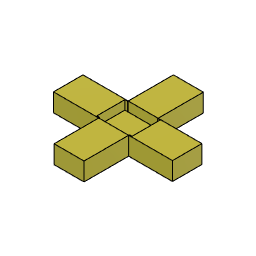
BMO_Joystick (Autodesk Fusion 360 design; units mm, degrees)
Autodesk Fusion 360 part; units mm, degrees
sketch "스케치1" plane through (0, 0, 0) normal (0, 1, 0) x (1, 0, 0)
  line L0 (5.2558, 0.4095) -> (68.4042, 0.4095)
  line L1 (73.4042, -4.5905) -> (73.4042, -43.5505)
  line L2 (0.2558, -43.5505) -> (0.2558, -4.5905)
  arc A0 (5.2558, 0.4095) -> (0.2558, -4.5905) centre (5.2558, -4.5905) ccw
  arc A1 (0.2558, -43.5505) -> (5.2558, -48.5505) centre (5.2558, -43.5505) ccw
  arc A2 (73.4042, -4.5905) -> (68.4042, 0.4095) centre (68.4042, -4.5905) ccw
  arc A3 (68.4259, -48.5505) -> (73.4042, -43.5505) centre (68.4042, -43.5505) ccw
  line L3 (8.0983, -61.4076) -> (32.8013, -61.4076)
  line L4 (32.8013, -61.4076) -> (32.8013, -65.2763)
  line L5 (32.8013, -65.2763) -> (8.0983, -65.2763)
  line L6 (8.0983, -65.2763) -> (8.0983, -61.4076)
  line L7 (33.6828, -66.6579) -> (7.2167, -66.6579)
  line L8 (6.7167, -66.1579) -> (6.7167, -60.526)
  line L9 (7.2167, -60.026) -> (33.6828, -60.026)
  line L10 (34.1828, -60.526) -> (34.1828, -66.1579)
  arc A4 (7.2167, -60.026) -> (6.7167, -60.526) centre (7.2167, -60.526) ccw
  arc A5 (6.7167, -66.1579) -> (7.2167, -66.6579) centre (7.2167, -66.1579) ccw
  arc A6 (34.1828, -60.526) -> (33.6828, -60.026) centre (33.6828, -60.526) ccw
  arc A7 (33.6828, -66.6579) -> (34.1828, -66.1579) centre (33.6828, -66.1579) ccw
  line L11 (19.1249, -96.9501) -> (32.2249, -96.9501)
  line L12 (32.2249, -96.9501) -> (32.2249, -102.6301)
  line L13 (32.2249, -102.6301) -> (19.1249, -102.6301)
  line L14 (19.1249, -102.6301) -> (19.1249, -96.9501)
  line L15 (3.6186, -96.8594) -> (16.7186, -96.8594)
  line L16 (16.7186, -96.8594) -> (16.7186, -102.5394)
  line L17 (16.7186, -102.5394) -> (3.6186, -102.5394)
  line L18 (3.6186, -102.5394) -> (3.6186, -96.8594)
  line L19 (-5.4373, 16.7169) -> (79.6514, 16.7169)
  line L20 (81.6514, 14.7169) -> (81.6514, -111.2831)
  line L21 (79.6514, -113.2831) -> (-5.4373, -113.2831)
  line L22 (-7.4373, -111.2831) -> (-7.4373, 14.7169)
  line L23 (12.7325, -76.8859) -> (16.6325, -76.8859)
  line L24 (16.6325, -76.8859) -> (16.6325, -79.9859)
  line L25 (16.6325, -79.9859) -> (12.7325, -79.9859)
  line L26 (12.7325, -79.9859) -> (12.7325, -76.8859)
  circle A8 centre (57.8034, -66.7955) radius 7
  circle A9 centre (56.6109, -95.955) radius 13.4
  circle A10 centre (56.6109, -95.955) radius 12
  line L27 (13.0415, -71.8299) -> (16.3471, -71.8299)
  line L28 (16.3471, -71.8299) -> (16.3471, -85.0178)
  line L29 (16.3471, -85.0178) -> (13.0415, -85.0178)
  line L30 (13.0415, -85.0178) -> (13.0415, -71.8299)
  line L31 (8.0415, -76.8299) -> (21.1916, -76.8299)
  line L32 (21.1916, -76.8299) -> (21.1916, -80.0863)
  line L33 (21.1916, -80.0863) -> (8.0415, -80.0863)
  line L34 (8.0415, -80.0863) -> (8.0415, -76.8299)
  line L35 (6.7208, -81.407) -> (6.7208, -75.5092)
  line L36 (6.7208, -75.5092) -> (22.5123, -75.5092)
  line L37 (22.5123, -75.5092) -> (22.5123, -81.407)
  line L38 (22.5123, -81.407) -> (6.7208, -81.407)
  line L39 (11.7155, -86.3438) -> (11.7155, -70.5039)
  line L40 (11.7155, -70.5039) -> (17.6731, -70.5039)
  line L41 (17.6731, -70.5039) -> (17.6731, -86.3438)
  line L42 (17.6731, -86.3438) -> (11.7155, -86.3438)
  arc A11 (-5.4373, 16.7169) -> (-7.4373, 14.7169) centre (-5.4373, 14.7169) ccw
  arc A12 (-3.4468, 14.3074) -> (-5.4468, 12.3074) centre (-3.4468, 12.3074) ccw
  arc A13 (81.6514, 14.7169) -> (79.6514, 16.7169) centre (79.6514, 14.7169) ccw
  arc A14 (79.6419, 12.3074) -> (77.6419, 14.3074) centre (77.6419, 12.3074) ccw
  arc A15 (-7.4373, -111.2831) -> (-5.4373, -113.2831) centre (-5.4373, -111.2831) ccw
  arc A16 (-5.4468, -102.8328) -> (-3.4468, -104.8328) centre (-3.4468, -102.8328) ccw
  arc A17 (77.6419, -104.8328) -> (79.6419, -102.8328) centre (77.6419, -102.8328) ccw
  arc A18 (79.6514, -113.2831) -> (81.6514, -111.2831) centre (79.6514, -111.2831) ccw
  line L43 (79.6514, 14.7169) -> (79.6514, -111.2831)
  line L44 (-5.4373, 14.7169) -> (79.6514, 14.7169)
  line L45 (-5.4373, -111.2831) -> (-5.4373, 14.7169)
  line L46 (79.6514, -111.2831) -> (-5.4373, -111.2831)
  line L47 (42.3168, -54.3547) -> (72.3168, -54.3547)
  line L48 (72.3168, -54.3547) -> (72.3168, -79.8547)
  line L49 (72.3168, -79.8547) -> (42.3168, -79.8547)
  line L50 (42.3168, -79.8547) -> (42.3168, -54.3547)
  arc A19 (-1.2442, -43.5505) -> (5.2558, -50.0505) centre (5.2558, -43.5505) ccw
  line L51 (-1.2442, -43.5505) -> (-1.2442, -4.5905)
  arc A20 (5.2558, 1.9095) -> (-1.2442, -4.5905) centre (5.2558, -4.5905) ccw
  line L52 (5.2558, 1.9095) -> (68.4042, 1.9095)
  arc A21 (74.9042, -4.5905) -> (68.4042, 1.9095) centre (68.4042, -4.5905) ccw
  line L53 (74.9042, -4.5905) -> (74.9042, -43.5505)
  arc A22 (68.4323, -50.0505) -> (74.9042, -43.5505) centre (68.4042, -43.5505) ccw
  line L54 (5.2558, -50.0505) -> (68.4323, -50.0505)
  line L55 (5.2558, -48.5505) -> (68.4259, -48.5505)
  line L56 (-3.5681, -64.3856) -> (30.2319, -64.3856)
  line L57 (30.2319, -64.3856) -> (30.2319, -91.3856)
  line L58 (30.2319, -91.3856) -> (-3.5681, -91.3856)
  line L59 (-3.5681, -91.3856) -> (-3.5681, -64.3856)
  line L60 (3.782, -65.3602) -> (24.782, -65.3602)
  line L61 (24.782, -65.3602) -> (24.782, -91.2602)
  line L62 (24.782, -91.2602) -> (3.782, -91.2602)
  line L63 (3.782, -91.2602) -> (3.782, -65.3602)
  point P0 (-7.4373, 16.7169)
  point P1 (81.6514, 16.7169)
  point P2 (81.6514, -113.2831)
  point P3 (-5.4468, 14.3074)
  point P4 (79.6419, 14.3074)
  point P5 (79.6419, -104.8328)
  dimension "d3" = 5
  dimension "d4" = 5
  dimension "d5" = 5
  dimension "d6" = 5
  dimension "d10" = 0.5
  dimension "d11" = 0.5
  dimension "d12" = 0.5
  dimension "d13" = 0.5
  dimension "d14" = 13.1
  dimension "d15" = 5.68
  dimension "d16" = 13.1
  dimension "d17" = 5.68
  dimension "d20" = 89.0887
  dimension "d21" = 130
  dimension "d22" = 85.0887
  dimension "d23" = 119.1403
  dimension "d24" = 26.4662
  dimension "d25" = 5.6319
  dimension "d26" = 24.703
  dimension "d27" = 3.8687
  dimension "d28" = 63.1484
  dimension "d29" = 38.96
  dimension "d32" = 3.9
  dimension "d33" = 3.1
  dimension "d34" = 14
  dimension "d35" = 26.8
  dimension "d36" = 24
  dimension "d37" = -1.3207
  dimension "d38" = -1.326
  dimension "d39" = 13.1501
  dimension "d40" = 15.7915
  dimension "d41" = 3.3056
  dimension "d42" = 15.8399
  dimension "d43" = 13.1879
  dimension "d44" = 3.2564
  dimension "d45" = 5.8978
  dimension "d46" = 2
  dimension "d47" = 2
  dimension "d48" = 2
  dimension "d49" = 2
  dimension "d50" = 2
  dimension "d51" = 2
  dimension "d52" = 2
  dimension "d53" = 2
  dimension "d54" = 14.8074
  dimension "d57" = 2
  dimension "d95" = 30
  dimension "d96" = 25.5
  dimension "d119" = 33.8
  dimension "d120" = 27
  dimension "d121" = 21
  dimension "d122" = 25.9
  constraint horizontal L0
  constraint vertical L1
  constraint vertical L2
  constraint tangent L2 A0
  constraint tangent L0 A0
  constraint tangent L2 A1
  constraint tangent L1 A2
  constraint tangent L0 A2
  constraint tangent L1 A3
  constraint horizontal L3
  constraint vertical L4
  constraint horizontal L5
  constraint vertical L6
  constraint parallel L5 L7
  constraint parallel L6 L8
  constraint parallel L3 L9
  constraint parallel L4 L10
  constraint tangent L8 A4
  constraint tangent L9 A4
  constraint tangent L8 A5
  constraint tangent L7 A5
  constraint tangent L9 A6
  constraint tangent L10 A6
  constraint tangent L10 A7
  constraint tangent L7 A7
  constraint horizontal L11
  constraint vertical L12
  constraint horizontal L13
  constraint vertical L14
  constraint horizontal L15
  constraint vertical L16
  constraint horizontal L17
  constraint vertical L18
  constraint horizontal L19
  constraint vertical L20
  constraint horizontal L21
  constraint vertical L22
  constraint horizontal L23
  constraint vertical L24
  constraint horizontal L25
  constraint vertical L26
  constraint concentric A9 A10
  constraint horizontal L27
  constraint vertical L28
  constraint horizontal L29
  constraint vertical L30
  constraint horizontal L31
  constraint vertical L32
  constraint horizontal L33
  constraint vertical L34
  constraint coincident P0 L22
  constraint coincident P0 L19
  constraint tangent L22 A11
  constraint tangent L19 A11
  constraint coincident P1 L19
  constraint coincident P1 L20
  constraint tangent L19 A13
  constraint tangent L20 A13
  constraint tangent L22 A15
  constraint tangent L21 A15
  constraint coincident P2 L20
  constraint coincident P2 L21
  constraint tangent L20 A18
  constraint tangent L21 A18
  constraint horizontal L47
  constraint vertical L48
  constraint horizontal L49
  constraint vertical L50
  constraint concentric A1 A19
  constraint parallel L2 L51
  constraint concentric A0 A20
  constraint parallel L0 L52
  constraint concentric A2 A21
  constraint parallel L1 L53
  constraint concentric A3 A22
  constraint tangent L52 A21
  constraint tangent A19 L51
  constraint tangent L53 A22
  constraint tangent A21 L53
  constraint tangent L51 A20
  constraint tangent A20 L52
  constraint horizontal L56
  constraint vertical L57
  constraint horizontal L58
  constraint vertical L59
  constraint horizontal L60
  constraint vertical L61
  constraint horizontal L62
  constraint vertical L63
  measures "d3" radius of A0
  measures "d4" radius of A1
  measures "d5" radius of A2
  measures "d6" radius of A3
  measures "d10" radius of A4
  measures "d11" radius of A5
  measures "d12" radius of A6
  measures "d13" radius of A7
  measures "d14" distance of L11.start L11.end
  measures "d15" distance of L11.start L13.end
  measures "d16" distance of L15.start L15.end
  measures "d17" distance of L15.start L17.end
  measures "d20" distance of P0 P1
  measures "d21" distance of P1 P2
  measures "d22" distance of P3 P4
  measures "d23" distance of P4 P5
  measures "d24" distance of L9.start L9.end
  measures "d25" distance of L10.start L10.end
  measures "d26" distance of L3.start L3.end
  measures "d27" distance of L3.end L4.end
  measures "d28" distance of A20.start L52.end
  measures "d29" distance of A21.start L53.end
  measures "d32" distance of L23.start L23.end
  measures "d33" distance of L23.start L25.end
  measures "d34" diameter of A8
  measures "d35" diameter of A9
  measures "d36" diameter of A10
  measures "d39" distance of L31.start L31.end
  measures "d40" distance of L35.end L36.end
  measures "d41" distance of L27.start L27.end
  measures "d42" distance of L39.start L39.end
  measures "d43" distance of L27.start L29.end
  measures "d44" distance of L31.start L33.end
  measures "d45" distance of L35.start L35.end
  measures "d46" radius of A11
  measures "d47" radius of A12
  measures "d48" radius of A13
  measures "d49" radius of A14
  measures "d50" radius of A15
  measures "d51" radius of A16
  measures "d52" radius of A17
  measures "d53" radius of A18
  measures "d54" distance of L19 L52
  measures "d95" distance of L48.end L49.end
  measures "d96" distance of L47.end L48.end
  measures "d119" distance of L56.start L56.end
  measures "d120" distance of L56.start L58.end
  measures "d121" distance of L60.start L60.end
  measures "d122" distance of L60.start L62.end
sketch "스케치2" plane through (286.6514, 0, 0) normal (1, 0, 0) x (0, 0, -1)
  line L0 (-111.2831, 0) -> (14.7169, 0)
  line L1 (14.7169, 0) -> (14.7169, 30)
  line L2 (14.7169, 30) -> (-111.2831, 30)
  line L3 (-111.2831, 30) -> (-111.2831, 0)
  line L4 (-87.1899, 4.8048) -> (5.0207, 5.1018) construction
  line L5 (5.0207, 5.1018) -> (4.9496, 27.1657) construction
  line L6 (4.9496, 27.1657) -> (-87.261, 26.8686) construction
  line L7 (-87.261, 26.8686) -> (-87.1899, 4.8048) construction
  circle A0 centre (-98, 14) radius 1
  circle A1 centre (-94.5923, 21.5266) radius 1
  circle A2 centre (-105.6179, 15.0752) radius 1
  circle A3 centre (-101.4738, 8.3604) radius 1
  circle A4 centre (-93.909, 8.4262) radius 1
  circle A5 centre (-91.1462, 14.9435) radius 1
  circle A6 centre (-101.408, 21) radius 1
  dimension "d74" = 25
  dimension "d84" = 2
  dimension "d85" = 2
  dimension "d87" = 2
  dimension "d88" = 2
  dimension "d89" = 2
  dimension "d90" = 2
  dimension "d91" = 2
  measures "d84" diameter of A0
  measures "d85" diameter of A1
  measures "d87" diameter of A2
  measures "d88" diameter of A3
  measures "d89" diameter of A4
  measures "d90" diameter of A5
  measures "d91" diameter of A6
sketch "스케치3" plane through (197.5627, 0, 0) normal (-1, 0, 0) x (0, 0, 1)
  line L0 (-14.7169, 0) -> (111.2831, 0)
  line L1 (111.2831, 0) -> (111.2831, 30)
  line L2 (111.2831, 30) -> (-14.7169, 30)
  line L3 (-14.7169, 30) -> (-14.7169, 0)
  line L4 (7.2946, 2.9984) -> (75.3904, 3.0024) construction
  line L5 (75.3904, 3.0024) -> (75.389, 27.1757) construction
  line L6 (75.389, 27.1757) -> (7.2931, 27.1717) construction
  line L7 (7.2931, 27.1717) -> (7.2946, 2.9984) construction
  dimension "d77" = 25
sketch "스케치4" plane through (0, 2, 0) normal (0, 1, 0) x (-1, 0, 0)
  arc A0 (-92.5627, 111.2831) -> (-94.5627, 113.2831) centre (-94.5627, 111.2831) ccw
  line L0 (-94.5627, 113.2831) -> (-179.6514, 113.2831)
  arc A1 (-179.6514, 113.2831) -> (-181.6514, 111.2831) centre (-179.6514, 111.2831) ccw
  line L1 (-181.6514, 111.2831) -> (-181.6514, -14.7169)
  arc A2 (-181.6514, -14.7169) -> (-179.6514, -16.7169) centre (-179.6514, -14.7169) ccw
  line L2 (-179.6514, -16.7169) -> (-94.5627, -16.7169)
  arc A3 (-94.5627, -16.7169) -> (-92.5627, -14.7169) centre (-94.5627, -14.7169) ccw
  line L3 (-92.5627, -14.7169) -> (-92.5627, 111.2831)
  line L4 (-104.1542, -7.6516) -> (-110, -7.6516)
  line L5 (-110, -7.6516) -> (-110, 25)
  line L6 (-110, 25) -> (-104.1542, 25)
  line L7 (-104.1542, 25) -> (-104.1542, -7.6516)
  line L8 (-126, -7.6516) -> (-126, 25)
  line L9 (-120.1542, 25) -> (-120.1542, -7.6516)
  line L10 (-126, 25) -> (-120.1542, 25)
  line L11 (-120.1542, -7.6516) -> (-126, -7.6516)
  line L12 (-141, -7.6516) -> (-141, 25)
  line L13 (-135.1542, 25) -> (-135.1542, -7.6516)
  line L14 (-141, 25) -> (-135.1542, 25)
  line L15 (-135.1542, -7.6516) -> (-141, -7.6516)
  line L16 (-156, -7.6516) -> (-156, 25)
  line L17 (-150.1542, 25) -> (-150.1542, -7.6516)
  line L18 (-156, 25) -> (-150.1542, 25)
  line L19 (-150.1542, -7.6516) -> (-156, -7.6516)
  line L20 (-171, -7.6516) -> (-171, 25)
  line L21 (-165.1542, 25) -> (-165.1542, -7.6516)
  line L22 (-171, 25) -> (-165.1542, 25)
  line L23 (-165.1542, -7.6516) -> (-171, -7.6516)
  line L24 (-107.3831, 39.4897) -> (-170, 39.4897)
  line L25 (-170, 39.4897) -> (-170, 90)
  line L26 (-170, 90) -> (-107.3831, 90)
  line L27 (-107.3831, 90) -> (-107.3831, 39.4897)
  constraint horizontal L4
  constraint vertical L5
  constraint horizontal L6
  constraint vertical L7
  constraint horizontal L11
  constraint vertical L8
  constraint horizontal L10
  constraint vertical L9
  constraint horizontal L15
  constraint vertical L12
  constraint horizontal L14
  constraint vertical L13
  constraint horizontal L19
  constraint vertical L16
  constraint horizontal L18
  constraint vertical L17
  constraint horizontal L23
  constraint vertical L20
  constraint horizontal L22
  constraint vertical L21
  constraint horizontal L24
  constraint vertical L25
  constraint horizontal L26
  constraint vertical L27
sketch "스케치5" plane through (0, 0, 0) normal (0, 1, 0) x (1, 0, 0)
  circle A0 centre (43.9407, -55.8888) radius 1.5
  circle A1 centre (70.9407, -55.8888) radius 1.5
  circle A2 centre (43.9407, -78.8888) radius 1.5
  circle A3 centre (70.9407, -78.8888) radius 1.5
  circle A4 centre (28, -89) radius 2
  circle A5 centre (28, -66) radius 2
  circle A6 centre (-2, -89) radius 2
  circle A7 centre (-2, -65) radius 2
  dimension "d109" = 3
  dimension "d110" = 3
  dimension "d111" = 3
  dimension "d112" = 3
  dimension "d123" = 4
  dimension "d124" = 4
  dimension "d125" = 4
  dimension "d126" = 4
  measures "d109" diameter of A0
  measures "d110" diameter of A1
  measures "d111" diameter of A2
  measures "d112" diameter of A3
  measures "d123" diameter of A4
  measures "d124" diameter of A5
  measures "d125" diameter of A6
  measures "d126" diameter of A7
extrude "돌출23" add sketch "스케치1" along normal blind 1 contours L23 L25 L26 L30 | L23 L25 L28 L30 | L23 L24 L25 L28 makes body 1
extrude "돌출24" add sketch "스케치1" along normal blind 2 separate body contours L23 L25 L26 L30 L31 L33 L39 | L23 L24 L25 L28 L31 L33 L41 | L28 L30 L31 L36 | L28 L30 L33 L38 | L27 L28 L30 L36 | L31 L33 L34 L39 | L31 L32 L33 L41 | L28 L29 L30 L38 makes body 2 at (9.6052, 0, 78.9673)
move_body "이동15" bodies 2 1 to x (1, 0, 0) y (0, 1, 0) z (0, 0, 1) at (-200, 0, -50)
extrude "돌출20" [suppressed]
move_body "이동9" [suppressed]
